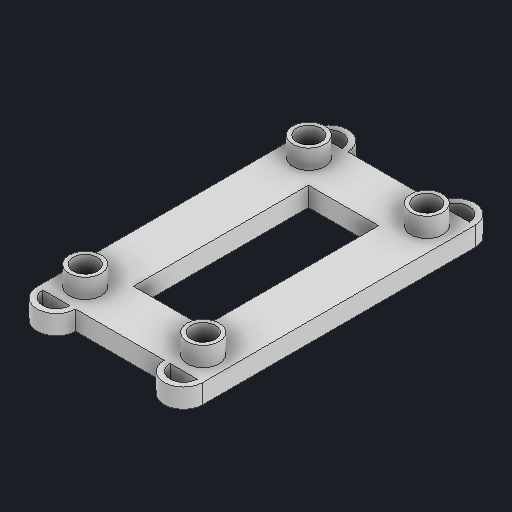
# Autodesk Inventor part: carriage_top
Saved by Autodesk Inventor 2025 (Build 290162010, 162A)
## iProperties
Created: 2024-06-21
Part Number: carriage_top
Material: Generic
Document SubType Name: Modeling
Designer: mihir
Density: 1 g/cm^3
Appearance: Default
Author: mihir
Autodesk Inventor part; units mm, degrees
ref_plane "YZ Plane" through (0, 0, 0) normal (1, 0, 0) x (0, 1, 0)
ref_plane "XZ Plane" through (0, 0, 0) normal (0, 1, 0) x (-1, 0, 0)
ref_plane "XY Plane" through (0, 0, 0) normal (0, 0, 1) x (1, 0, 0)
sketch "Sketch1" plane through (0, 0, 0) normal (0, 1, 0) x (-1, 0, 0)
  line L0 (0, 0) -> (43, 0)
  line L1 (43, 0) -> (43, -70.6)
  line L2 (43, -70.6) -> (0, -70.6)
  line L3 (0, -70.6) -> (0, 0)
  line L4 (12.4, -12.6) -> (30.6, -12.6)
  line L5 (30.6, -12.6) -> (30.6, -58)
  line L6 (30.6, -58) -> (12.4, -58)
  line L7 (12.4, -58) -> (12.4, -12.6)
  line L8 (30.6, -35.3) -> (43, -35.3) construction
  line L9 (21.5, -12.6) -> (21.5, 0) construction
  arc A0 (43, 0) -> (33, 0) centre (38, 0) ccw
  arc A1 (10, 0) -> (0, 0) centre (5, 0) ccw
  arc A2 (41.5, 0) -> (34.5, 0) centre (38, 0) ccw
  arc A3 (8.5, 0) -> (1.5, 0) centre (5, 0) ccw
  arc A4 (33, -70.6) -> (43, -70.6) centre (38, -70.6) ccw
  arc A5 (0, -70.6) -> (10, -70.6) centre (5, -70.6) ccw
  arc A6 (34.5, -70.6) -> (41.5, -70.6) centre (38, -70.6) ccw
  arc A7 (1.5, -70.6) -> (8.5, -70.6) centre (5, -70.6) ccw
  point P0 (41.5, -70.6)
  dimension "d0" = 70.6
  dimension "d1" = 43
  dimension "d2" = 45.4
  dimension "d3" = 18.2
  dimension "d4" = 5
  dimension "d5" = 5
  dimension "d6" = 1.5
  dimension "d7" = 1.5
  constraints: 18 end point, 16 point on circle, 10 symmetric about line, 8 centre point, 4 coincident, 3 horizontal, 3 midpoint, 3 parallel, 2 tangent, 2 vertical, 1 perpendicular, 14 other
  measures "d0" distance of L2.end L3.end
  measures "d1" distance of L3.end L1.start
  measures "d2" distance of L6.end L4.start
  measures "d3" distance of L5.end L6.end
  measures "d4" radius of A0
  measures "d5" radius of A1
  measures "d6" radial gap between concentric circles of A0 A2
  measures "d7" radial gap between concentric circles of A1 A3
extrude "Extrusion1" add sketch "Sketch1" along normal blind 5 contours A1 L0 A3 | L0 L1 L2 L3 | L2 A7 A5 | A0 L0 A2 | L2 A6 A4
sketch "Sketch2" plane through (0, 5, 0) normal (0, 1, 0) x (1, 0, 0)
  line L0 (-33, 0) -> (-10, 0) construction
  line L1 (-12.4, 58) -> (-12.4, 12.6) construction
  line L2 (-10, 0) -> (-10, 12.6) construction
  line L3 (-12.4, 12.6) -> (-2.4, 12.6) construction
  line L4 (-12.4, 12.6) -> (0, 0) construction
  arc A0 (-10, 0) -> (0, 0) centre (-5, 0) ccw construction
  line L5 (-10, 0) -> (0, 0) construction
  line L6 (-5, 0) -> (-6.2, 6.3) construction
  line L7 (-43, 70.6) -> (-43, 0) construction
  line L8 (-43, 35.3) -> (0, 35.3) construction
  line L9 (0, 0) -> (0, 70.6) construction
  line L10 (-21.5, 0) -> (-21.5, 70.6) construction
  line L11 (-10, 70.6) -> (-33, 70.6) construction
  circle A1 centre (-6.2, 6.3) radius 3.15
  circle A2 centre (-6.2, 6.3) radius 4.15
  circle A3 centre (-6.2, 64.3) radius 3.15
  circle A4 centre (-6.2, 64.3) radius 4.15
  circle A5 centre (-36.8, 6.3) radius 3.15
  circle A6 centre (-36.8, 6.3) radius 4.15
  circle A7 centre (-36.8, 64.3) radius 3.15
  circle A8 centre (-36.8, 64.3) radius 4.15
  dimension "d10" = 1
  dimension "d11" = 6.3
  constraints: 14 end point, 8 centre point, 6 symmetric about line, 5 coincident, 4 midpoint, 1 horizontal, 1 parallel, 1 perpendicular, 8 other
  measures "d10" radial gap between concentric circles of A2 A1
  measures "d11" diameter of A1
extrude "Extrusion2" add sketch "Sketch2" along normal blind 5
equation "\"d0\" = carriage_top_length"
equation "\"d1\" = carriage_top_width"
equation "\"d2\" = carriage_mount_cutout_length"
equation "\"d3\" = carriage_mount_cutout_width"
equation "\"d8\" = carriage_top_thickness"
equation "\"d10\" = carriage_mount_wall_thickness"
equation "\"d11\" = rod_diameter + rod_tolerance"
equation "\"d12\" = carriage_top_thickness"
equation "\"carriage_mount_cutout_length\" = 45.4"
equation "\"carriage_mount_cutout_width\" = 18.2"
equation "\"carriage_top_length\" = 70.6"
equation "\"carriage_top_width\" = 43"
equation "\"carriage_top_thickness\" = 5"
equation "\"carriage_mount_wall_thickness\" = 1"
equation "\"rod_diameter\" = 6"
equation "\"rod_tolerance\" = 0.3"
body "Solid1"
